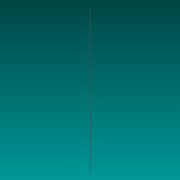
# Autodesk Inventor part: 8907K48 045 Phosphate Rod
Saved by Autodesk Inventor 2015 (Build 190159000, 159)
## iProperties
Created: 2014-10-17
Part Number: 8907K48 045 Phosphate Rod
Material: Steel, Carbon
Document SubType Name: Modeling
Designer: Sawaiz Syed
Density: 7.85 g/cm^3
Appearance: Semi-Polished
Author: Sawaiz Syed
Autodesk Inventor part; units mm, degrees
ref_plane "YZ Plane" through (0, 0, 0) normal (1, 0, 0) x (0, 1, 0)
ref_plane "XZ Plane" through (0, 0, 0) normal (0, 1, 0) x (-1, 0, 0)
ref_plane "XY Plane" through (0, 0, 0) normal (0, 0, 1) x (1, 0, 0)
sketch "Sketch1" plane through (0, 0, 0) normal (0, 0, 1) x (1, 0, 0)
  circle A0 centre (0, 0) radius 0.5715
  dimension "d0" = 1.143
  constraints: 1 centre point, 1 coincident
  measures "d0" diameter of A0
extrude "Extrusion1" add sketch "Sketch1" along normal mid plane 304.8
body "Solid1"
